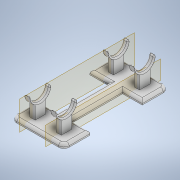
# Autodesk Inventor part: support
Saved by Autodesk Inventor 2022 (Build 260153000, 153)
## iProperties
Created: 2023-01-14
Part Number: support
Material: Generic
Document SubType Name: Modeling
Designer: zhong
Density: 1 g/cm^3
Appearance: Default
Author: zhong
Autodesk Inventor part; units mm, degrees
ref_plane "XZ Plane" through (0, 0, 0) normal (0, 1, 0) x (-1, 0, 0)
ref_plane "XY Plane" through (0, 0, 0) normal (0, 0, 1) x (1, 0, 0)
sketch "Sketch1" plane through (0, 0, 0) normal (0, 1, 0) x (-1, 0, 0)
  line L0 (-80, -200) -> (80, -200)
  line L1 (100, -180) -> (100, 180)
  line L2 (80, 200) -> (-80, 200)
  line L3 (-100, 180) -> (-100, -180)
  line L4 (-100, -200) -> (100, 200) construction
  line L5 (100, -200) -> (-100, 200) construction
  arc A0 (100, 180) -> (80, 200) centre (80, 180) ccw
  arc A1 (80, -200) -> (100, -180) centre (80, -180) ccw
  arc A2 (-100, -180) -> (-80, -200) centre (-80, -180) ccw
  arc A3 (-80, 200) -> (-100, 180) centre (-80, 180) ccw
  point P0 (0, 0)
  dimension "d0" = 200
  dimension "d1" = 400
  dimension "d2" = 20
  constraints: 12 end point, 8 point on circle, 8 point on line, 8 tangent, 4 centre point, 3 equal radius, 2 midpoint, 2 parallel, 1 horizontal, 1 perpendicular
  measures "d0" distance of L5.end L4.end
  measures "d1" distance of L4.end L5.start
  measures "d2" radius of A0
extrude "Extrusion1" add sketch "Sketch1" along normal blind 15
sketch "Sketch3" plane through (0, 15, 0) normal (0, 1, 0) x (1, 0, 0)
  line L0 (-100, 180) -> (-100, -180) projected
  line L1 (-100, -100) -> (-25, -100)
  line L2 (-25, -100) -> (-25, 100)
  line L3 (-25, 100) -> (-100, 100)
  line L4 (-100, 100) -> (-100, -100)
  line L5 (100, -180) -> (100, 180) projected
  line L6 (100, -100) -> (25, -100)
  line L7 (25, -100) -> (25, 100)
  line L8 (25, 100) -> (100, 100)
  line L9 (100, 100) -> (100, -100)
  point P0 (0, 0)
  dimension "d5" = 75
  dimension "d6" = 200
  dimension "d7" = 75
  constraints: 16 end point, 4 parallel, 4 point on line, 2 horizontal, 2 perpendicular
  measures "d5" distance of L3.end L2.end
  measures "d6" distance of L2.end L1.end
  measures "d7" distance of L7.end L8.end
extrude "Extrusion2" cut sketch "Sketch3" against normal blind 15
fillet "Fillet1" radius 10 16 edges at (-62.5, 15, 100) (62.5, 15, 100) (62.5, 15, -100) (-62.5, 15, -100) (-25, 15, 0) (25, 15, 0) (-94.1421, 15, -194.1421) (0, 15, -200) (94.1421, 15, -194.1421) (100, 15, -140) (-100, 15, -140) (-94.1421, 15, 194.1421) (0, 15, 200) (94.1421, 15, 194.1421) (100, 15, 140) (-100, 15, 140)
sketch "Sketch5" plane through (0, 15, 0) normal (0, 1, 0) x (1, 0, 0)
  line L0 (40, -170) -> (60, -170)
  line L1 (60, -170) -> (60, -130)
  line L2 (60, -130) -> (40, -130)
  line L3 (40, -130) -> (40, -170)
  line L4 (40, -170) -> (60, -130) construction
  line L5 (60, -170) -> (40, -130) construction
  line L6 (-60, -170) -> (-40, -170)
  line L7 (-40, -170) -> (-40, -130)
  line L8 (-40, -130) -> (-60, -130)
  line L9 (-60, -130) -> (-60, -170)
  line L10 (-60, -170) -> (-40, -130) construction
  line L11 (-40, -170) -> (-60, -130) construction
  line L12 (40, 130) -> (60, 130)
  line L13 (60, 130) -> (60, 170)
  line L14 (60, 170) -> (40, 170)
  line L15 (40, 170) -> (40, 130)
  line L16 (40, 130) -> (60, 170) construction
  line L17 (60, 130) -> (40, 170) construction
  line L18 (-60, 130) -> (-40, 130)
  line L19 (-40, 130) -> (-40, 170)
  line L20 (-40, 170) -> (-60, 170)
  line L21 (-60, 170) -> (-60, 130)
  line L22 (-60, 130) -> (-40, 170) construction
  line L23 (-40, 130) -> (-60, 170) construction
  point P0 (0, 0)
  point P1 (50, -150)
  point P2 (-50, -150)
  point P3 (50, 150)
  point P4 (-50, 150)
  dimension "d11" = 20
  dimension "d12" = 40
  dimension "d13" = 40
  constraints: 48 end point, 8 midpoint, 8 parallel, 4 horizontal, 4 perpendicular, 4 point on line
  measures "d11" distance of L2.end L1.end
  measures "d12" distance of L1.end L0.end
  measures "d13" distance of L13.end L12.end
extrude "Extrusion3" add sketch "Sketch5" along normal blind 50
ref_plane "Work Plane1" through (50, 0, 0) normal (1, 0, 0) x (0, 1, 0)
sketch "Sketch6" plane through (50, 0, 0) normal (1, 0, 0) x (0, 1, 0)
  line L0 (15, 130) -> (65, 130) projected
  arc A0 (100, 190.3113) -> (100, 109.6887) centre (100, 150) ccw
  arc A1 (100, 185) -> (100, 115) centre (100, 150) ccw
  line L1 (100, 115) -> (100, 109.6887)
  line L2 (100, 185) -> (100, 190.3113)
  line L3 (65, -130) -> (65, -170) projected
  arc A2 (100, -109.6887) -> (100, -190.3113) centre (100, -150) ccw
  arc A3 (100, -115) -> (100, -185) centre (100, -150) ccw
  line L4 (100, -185) -> (100, -190.3113)
  line L5 (100, -115) -> (100, -109.6887)
  point P0 (0, 0)
  constraints: 10 point on circle, 8 end point, 4 centre point, 2 coincident, 2 point on line, 2 vertical
extrude "Extrusion4" add sketch "Sketch6" along normal mid plane 20
ref_plane "Work Plane2" through (-50, 0, 0) normal (1, 0, 0) x (0, 1, 0)
sketch "Sketch7" plane through (-50, 0, 0) normal (1, 0, 0) x (0, 1, 0)
  line L0 (15, -130) -> (65, -130) projected
  arc A0 (100, -109.6887) -> (100, -190.3113) centre (100, -150) ccw
  arc A1 (100, -115) -> (100, -185) centre (100, -150) ccw
  arc A2 (100, -109.6887) -> (65, -130) centre (100, -150) ccw projected
  line L1 (100, -115) -> (100, -109.6887)
  arc A3 (65, -170) -> (100, -190.3113) centre (100, -150) ccw projected
  line L2 (100, -185) -> (100, -190.3113)
  line L3 (65, 170) -> (65, 130) projected
  arc A4 (100, 190.3113) -> (100, 109.6887) centre (100, 150) ccw
  arc A5 (100, 185) -> (100, 115) centre (100, 150) ccw
  line L4 (100, 190.3113) -> (100, 185) projected
  line L5 (100, 185) -> (100, 190.3113)
  line L6 (100, 115) -> (100, 109.6887) projected
  line L7 (100, 115) -> (100, 109.6887)
  point P0 (0, 0)
  constraints: 10 point on circle, 8 end point, 4 centre point, 4 vertical, 2 coincident
extrude "Extrusion5" add sketch "Sketch7" along normal mid plane 20
fillet "Fillet2" radius 5 8 edges at (-50, 100, -185) (50, 100, -185) (50, 100, -115) (-50, 100, -115) (50, 100, 115) (-50, 100, 115) (50, 100, 185) (-50, 100, 185)
fillet "Fillet3" radius 5 24 edges at (40, 100, -189.9988) (40, 100, -110.0012) (40, 65, -150) (60, 100, -110.0012) (60, 100, -189.9988) (60, 65, -150) (-40, 100, -110.0012) (-40, 100, -189.9988) (-40, 65, -150) (-60, 100, -189.9988) (-60, 100, -110.0012) (-60, 65, -150) (-60, 100, 110.0012) (-60, 100, 189.9988) (-60, 65, 150) (-40, 100, 189.9988) (-40, 100, 110.0012) (-40, 65, 150) (40, 100, 110.0012) (40, 100, 189.9988) (40, 65, 150) (60, 100, 189.9988) (60, 100, 110.0012) (60, 65, 150)
body "Solid1"
